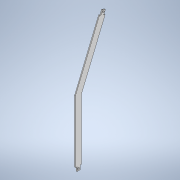
# Autodesk Inventor part: MotorSupport
Saved by Autodesk Inventor 2020 (Build 240168000, 168)
## iProperties
Created: 2019-06-18
Part Number: MotorSupport
Material: Generic
Document SubType Name: Modeling
Designer: Vivek Muskan
Density: 1 g/cm^3
Appearance: Default
Author: Vivek Muskan
Autodesk Inventor part; units mm, degrees
ref_plane "YZ Plane" through (0, 0, 0) normal (1, 0, 0) x (0, 1, 0)
ref_plane "XZ Plane" through (0, 0, 0) normal (0, 1, 0) x (-1, 0, 0)
ref_plane "XY Plane" through (0, 0, 0) normal (0, 0, 1) x (1, 0, 0)
sketch "Sketch2" plane through (0, 0, 0) normal (1, 0, 0) x (0, 1, 0)
  line L0 (0, 4) -> (60, 4)
  line L1 (0, 0) -> (60, 0)
  line L2 (0, -61) -> (0, 14)
  line L3 (96.4802, -36) -> (98.4802, -26)
  line L4 (96.4802, -36) -> (110.2083, 32.6406)
  line L5 (0, 0) -> (103.6802, 0)
  line L6 (0, 0) -> (0, -10)
  line L7 (0, -10) -> (101.6802, -10)
  line L8 (0, 0) -> (0, -2.5)
  line L9 (0, -2.5) -> (-7, -2.5)
  line L10 (-7, -2.5) -> (-7, -7.5)
  line L11 (-7, -7.5) -> (0, -7.5)
  line L12 (0, -2.5) -> (-4, -2.5)
  line L13 (-4, -2.5) -> (-4, -5)
  circle A0 centre (-4, -5) radius 1.5
  line L14 (198.4235, -42.1847) -> (202.1158, -43.7232)
  line L15 (204.885, -44.877) -> (202.9619, -49.4924)
  line L16 (198.4235, -42.1847) -> (204.885, -44.877)
  line L17 (202.9619, -49.4924) -> (196.5004, -46.8001)
  circle A1 centre (201.1542, -46.0308) radius 1.5
  line L18 (199.385, -39.877) -> (195.5388, -49.1078)
  line L19 (199.385, -39.877) -> (144.0004, -16.8001)
  line L20 (195.5388, -49.1078) -> (101.6802, -10)
  line L21 (199.385, -39.877) -> (103.6802, 0)
  point P0 (0, -7.5)
  dimension "d10" = 70
  dimension "d11" = 10
  dimension "d12" = 2.5
  dimension "d13" = 7
  dimension "d14" = 5
  dimension "d15" = 4
  dimension "d16" = 2.5
  dimension "d17" = 3
  constraints: 44 end point, 10 point on line, 9 symmetric about line, 6 perpendicular, 2 centre point, 1 coincident, 1 other
  measures "d10" distance of L3.start L4.end
  measures "d11" distance of L1.start L6.end
  measures "d12" distance of L1.start L8.end
  measures "d13" distance of L8.end L9.end
  measures "d14" distance of L9.end L10.end
  measures "d15" distance of L8.end L12.end
  measures "d16" distance of L12.end L13.end
  measures "d17" diameter of A0
extrude "Extrusion2" add sketch "Sketch2" along normal blind 1.5
body "Solid2"
